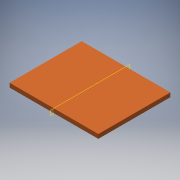
# Autodesk Inventor part: frontPlate
Saved by Autodesk Inventor 2016 SP1 (Build 200210100, 210)
## iProperties
Created: 2016-01-19
Part Number: frontPlate
Material: Wood (Walnut)
Document SubType Name: Modeling
Designer: steele
Density: 0.55 g/cm^3
Appearance: Walnut - Natural Polished
Author: steele
Autodesk Inventor part; units mm, degrees
ref_plane "XZ Plane" through (0, 0, 0) normal (0, 1, 0) x (-1, 0, 0)
ref_plane "XY Plane" through (0, 0, 0) normal (0, 0, 1) x (1, 0, 0)
sketch "Sketch1" plane through (0, 0, 0) normal (0, 1, 0) x (-1, 0, 0)
  line L0 (-203.2, 165.1) -> (-203.2, -165.1)
  line L1 (-203.2, -165.1) -> (203.2, -165.1)
  line L2 (203.2, -165.1) -> (203.2, 165.1)
  line L3 (203.2, 165.1) -> (-203.2, 165.1)
  line L4 (-203.2, 165.1) -> (203.2, -165.1) construction
  line L5 (-203.2, -165.1) -> (203.2, 165.1) construction
  point P0 (0, 0)
  dimension "d0" = 330.2
  dimension "d1" = 406.4
  constraints: 12 end point, 2 midpoint, 2 parallel, 1 perpendicular, 1 vertical
  measures "d0" distance of L1.end L2.end
  measures "d1" distance of L2.end L0.start
extrude "Extrusion1" add sketch "Sketch1" along normal blind 19.05
equation "\"d0\" = frontPlateLength"
equation "\"d1\" = frontPlateWidth"
equation "\"d2\" = frontPlateThickness"
equation "\"frontPlateWidth\" = 406.4"
equation "\"frontPlateLength\" = 330.2"
equation "\"frontPlateThickness\" = 19.05"
body "Solid1"
